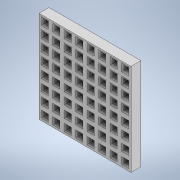
# Autodesk Inventor part: StandMatrix
Saved by Autodesk Inventor 2020.1 (Build 241239000, 239)
## iProperties
Created: 2019-09-02
Part Number: StandMatrix
Material: Generic
Document SubType Name: Modeling
Designer: matteo.spadetto-1
Density: 1 g/cm^3
Appearance: Default
Author: matteo.spadetto-1
Autodesk Inventor part; units mm, degrees
(part 1 of 2)
ref_plane "YZ Plane" through (0, 0, 0) normal (1, 0, 0) x (0, 1, 0)
ref_plane "XZ Plane" through (0, 0, 0) normal (0, 1, 0) x (-1, 0, 0)
ref_plane "XY Plane" through (0, 0, 0) normal (0, 0, 1) x (1, 0, 0)
sketch "Sketch1" plane through (0, 0, 0) normal (0, 0, 1) x (1, 0, 0)
  line L0 (1.062, 57.938) -> (1.062, 63.938)
  line L1 (1.062, 63.938) -> (7.062, 63.938)
  line L2 (7.062, 63.938) -> (7.062, 57.938)
  line L3 (7.062, 57.938) -> (1.062, 57.938)
  line L4 (17.31, 57.938) -> (23.31, 57.938)
  line L5 (23.31, 57.938) -> (23.31, 63.938)
  line L6 (23.31, 63.938) -> (17.31, 63.938)
  line L7 (17.31, 63.938) -> (17.31, 57.938)
  line L8 (9.186, 57.938) -> (15.186, 57.938)
  line L9 (15.186, 57.938) -> (15.186, 63.938)
  line L10 (15.186, 63.938) -> (9.186, 63.938)
  line L11 (9.186, 63.938) -> (9.186, 57.938)
  line L12 (25.434, 57.938) -> (31.434, 57.938)
  line L13 (31.434, 57.938) -> (31.434, 63.938)
  line L14 (31.434, 63.938) -> (25.434, 63.938)
  line L15 (25.434, 63.938) -> (25.434, 57.938)
  line L16 (33.558, 57.938) -> (39.558, 57.938)
  line L17 (39.558, 57.938) -> (39.558, 63.938)
  line L18 (39.558, 63.938) -> (33.558, 63.938)
  line L19 (33.558, 63.938) -> (33.558, 57.938)
  line L20 (47.682, 57.938) -> (41.682, 57.938)
  line L21 (41.682, 57.938) -> (41.682, 63.938)
  line L22 (41.682, 63.938) -> (47.682, 63.938)
  line L23 (47.682, 63.938) -> (47.682, 57.938)
  line L24 (55.806, 57.938) -> (49.806, 57.938)
  line L25 (49.806, 57.938) -> (49.806, 63.938)
  line L26 (49.806, 63.938) -> (55.806, 63.938)
  line L27 (55.806, 63.938) -> (55.806, 57.938)
  line L28 (63.93, 57.938) -> (57.93, 57.938)
  line L29 (57.93, 57.938) -> (57.93, 63.938)
  line L30 (57.93, 63.938) -> (63.93, 63.938)
  line L31 (63.93, 63.938) -> (63.93, 57.938)
  line L32 (1.062, 49.814) -> (1.062, 55.814)
  line L33 (1.062, 55.814) -> (7.062, 55.814)
  line L34 (7.062, 55.814) -> (7.062, 49.814)
  line L35 (7.062, 49.814) -> (1.062, 49.814)
  line L36 (9.186, 49.814) -> (15.186, 49.814)
  line L37 (15.186, 49.814) -> (15.186, 55.814)
  line L38 (15.186, 55.814) -> (9.186, 55.814)
  line L39 (9.186, 55.814) -> (9.186, 49.814)
  line L40 (17.31, 49.814) -> (17.31, 55.814)
  line L41 (17.31, 55.814) -> (23.31, 55.814)
  line L42 (23.31, 55.814) -> (23.31, 49.814)
  line L43 (23.31, 49.814) -> (17.31, 49.814)
  line L44 (25.434, 55.814) -> (31.434, 55.814)
  line L45 (31.434, 55.814) -> (31.434, 49.814)
  line L46 (31.434, 49.814) -> (25.434, 49.814)
  line L47 (33.558, 55.814) -> (39.558, 55.814)
  line L48 (39.558, 55.814) -> (39.558, 49.814)
  line L49 (39.558, 49.814) -> (33.558, 49.814)
  line L50 (47.682, 49.814) -> (41.682, 49.814)
  line L51 (41.682, 49.814) -> (41.682, 55.814)
  line L52 (41.682, 55.814) -> (47.682, 55.814)
  line L53 (47.682, 55.814) -> (47.682, 49.814)
  line L54 (49.806, 49.814) -> (55.806, 49.814)
  line L55 (55.806, 49.814) -> (55.806, 55.814)
  line L56 (55.806, 55.814) -> (49.806, 55.814)
  line L57 (49.806, 55.814) -> (49.806, 49.814)
  line L58 (63.93, 49.814) -> (57.93, 49.814)
  line L59 (57.93, 49.814) -> (57.93, 55.814)
  line L60 (57.93, 55.814) -> (63.93, 55.814)
  line L61 (63.93, 55.814) -> (63.93, 49.814)
  line L62 (1.062, 41.69) -> (7.062, 41.69)
  line L63 (7.062, 41.69) -> (7.062, 47.69)
  line L64 (7.062, 47.69) -> (1.062, 47.69)
  line L65 (1.062, 47.69) -> (1.062, 41.69)
  line L66 (9.186, 41.69) -> (9.186, 47.69)
  line L67 (9.186, 47.69) -> (15.186, 47.69)
  line L68 (15.186, 47.69) -> (15.186, 41.69)
  line L69 (15.186, 41.69) -> (9.186, 41.69)
  line L70 (23.31, 41.69) -> (23.31, 47.69)
  line L71 (23.31, 47.69) -> (17.31, 47.69)
  line L72 (17.31, 47.69) -> (17.31, 41.69)
  line L73 (17.31, 41.69) -> (23.31, 41.69)
  line L74 (31.434, 41.69) -> (25.434, 41.69)
  line L75 (25.434, 41.69) -> (25.434, 47.69)
  line L76 (25.434, 47.69) -> (31.434, 47.69)
  line L77 (31.434, 47.69) -> (31.434, 41.69)
  line L78 (39.558, 41.69) -> (33.558, 41.69)
  line L79 (33.558, 41.69) -> (33.558, 47.69)
  line L80 (33.558, 47.69) -> (39.558, 47.69)
  line L81 (39.558, 47.69) -> (39.558, 41.69)
  line L82 (47.682, 41.69) -> (47.682, 47.69)
  line L83 (47.682, 47.69) -> (41.682, 47.69)
  line L84 (41.682, 47.69) -> (41.682, 41.69)
  line L85 (41.682, 41.69) -> (47.682, 41.69)
  line L86 (55.806, 41.69) -> (55.806, 47.69)
  line L87 (55.806, 47.69) -> (49.806, 47.69)
  line L88 (49.806, 47.69) -> (49.806, 41.69)
  line L89 (49.806, 41.69) -> (55.806, 41.69)
  line L90 (63.93, 41.69) -> (63.93, 47.69)
  line L91 (63.93, 47.69) -> (57.93, 47.69)
  line L92 (57.93, 47.69) -> (57.93, 41.69)
  line L93 (57.93, 41.69) -> (63.93, 41.69)
  line L94 (7.062, 33.566) -> (1.062, 33.566)
  line L95 (1.062, 33.566) -> (1.062, 39.566)
  line L96 (1.062, 39.566) -> (7.062, 39.566)
  line L97 (7.062, 39.566) -> (7.062, 33.566)
  line L98 (15.186, 33.566) -> (15.186, 39.566)
  line L99 (15.186, 39.566) -> (9.186, 39.566)
  line L100 (9.186, 39.566) -> (9.186, 33.566)
  line L101 (9.186, 33.566) -> (15.186, 33.566)
  line L102 (17.31, 33.566) -> (23.31, 33.566)
  line L103 (23.31, 33.566) -> (23.31, 39.566)
  line L104 (23.31, 39.566) -> (17.31, 39.566)
  line L105 (17.31, 39.566) -> (17.31, 33.566)
  line L106 (25.434, 33.566) -> (31.434, 33.566)
  line L107 (31.434, 33.566) -> (31.434, 39.566)
  line L108 (31.434, 39.566) -> (25.434, 39.566)
  line L109 (25.434, 39.566) -> (25.434, 33.566)
  line L110 (39.558, 33.566) -> (33.558, 33.566)
  line L111 (33.558, 33.566) -> (33.558, 39.566)
  line L112 (33.558, 39.566) -> (39.558, 39.566)
  line L113 (39.558, 39.566) -> (39.558, 33.566)
  line L114 (41.682, 33.566) -> (41.682, 39.566)
  line L115 (41.682, 39.566) -> (47.682, 39.566)
  line L116 (47.682, 39.566) -> (47.682, 33.566)
  line L117 (47.682, 33.566) -> (41.682, 33.566)
  line L118 (55.806, 33.566) -> (49.806, 33.566)
  line L119 (49.806, 33.566) -> (49.806, 39.566)
  line L120 (49.806, 39.566) -> (55.806, 39.566)
  line L121 (55.806, 39.566) -> (55.806, 33.566)
  line L122 (63.93, 33.566) -> (57.93, 33.566)
  line L123 (57.93, 33.566) -> (57.93, 39.566)
  line L124 (57.93, 39.566) -> (63.93, 39.566)
  line L125 (63.93, 39.566) -> (63.93, 33.566)
  line L126 (25.434, 49.814) -> (25.434, 55.814)
  line L127 (33.558, 55.814) -> (33.558, 49.814)
  line L128 (1.062, 7.062) -> (1.062, 1.062)
  line L129 (1.062, 1.062) -> (7.062, 1.062)
  line L130 (7.062, 1.062) -> (7.062, 7.062)
  line L131 (7.062, 7.062) -> (1.062, 7.062)
  line L132 (17.31, 7.062) -> (23.31, 7.062)
  line L133 (23.31, 7.062) -> (23.31, 1.062)
  line L134 (23.31, 1.062) -> (17.31, 1.062)
  line L135 (17.31, 1.062) -> (17.31, 7.062)
  line L136 (9.186, 7.062) -> (15.186, 7.062)
  line L137 (15.186, 7.062) -> (15.186, 1.062)
  line L138 (15.186, 1.062) -> (9.186, 1.062)
  line L139 (9.186, 1.062) -> (9.186, 7.062)
  line L140 (25.434, 7.062) -> (31.434, 7.062)
  line L141 (31.434, 7.062) -> (31.434, 1.062)
  line L142 (31.434, 1.062) -> (25.434, 1.062)
  line L143 (25.434, 1.062) -> (25.434, 7.062)
  line L144 (33.558, 7.062) -> (39.558, 7.062)
  line L145 (39.558, 7.062) -> (39.558, 1.062)
  line L146 (39.558, 1.062) -> (33.558, 1.062)
  line L147 (33.558, 1.062) -> (33.558, 7.062)
  line L148 (47.682, 7.062) -> (41.682, 7.062)
  line L149 (41.682, 7.062) -> (41.682, 1.062)
  line L150 (41.682, 1.062) -> (47.682, 1.062)
  line L151 (47.682, 1.062) -> (47.682, 7.062)
  line L152 (55.806, 7.062) -> (49.806, 7.062)
  line L153 (49.806, 7.062) -> (49.806, 1.062)
  line L154 (49.806, 1.062) -> (55.806, 1.062)
  line L155 (55.806, 1.062) -> (55.806, 7.062)
  line L156 (63.93, 7.062) -> (57.93, 7.062)
  line L157 (57.93, 7.062) -> (57.93, 1.062)
  line L158 (57.93, 1.062) -> (63.93, 1.062)
  line L159 (63.93, 1.062) -> (63.93, 7.062)
  line L160 (1.062, 15.186) -> (1.062, 9.186)
  line L161 (1.062, 9.186) -> (7.062, 9.186)
  line L162 (7.062, 9.186) -> (7.062, 15.186)
  line L163 (7.062, 15.186) -> (1.062, 15.186)
  line L164 (9.186, 15.186) -> (15.186, 15.186)
  line L165 (15.186, 15.186) -> (15.186, 9.186)
  line L166 (15.186, 9.186) -> (9.186, 9.186)
  line L167 (9.186, 9.186) -> (9.186, 15.186)
  line L168 (17.31, 15.186) -> (17.31, 9.186)
  line L169 (17.31, 9.186) -> (23.31, 9.186)
  line L170 (23.31, 9.186) -> (23.31, 15.186)
  line L171 (23.31, 15.186) -> (17.31, 15.186)
  line L172 (25.434, 9.186) -> (31.434, 9.186)
  line L173 (31.434, 9.186) -> (31.434, 15.186)
  line L174 (31.434, 15.186) -> (25.434, 15.186)
  line L175 (33.558, 9.186) -> (39.558, 9.186)
  line L176 (39.558, 9.186) -> (39.558, 15.186)
  line L177 (39.558, 15.186) -> (33.558, 15.186)
  line L178 (47.682, 15.186) -> (41.682, 15.186)
  line L179 (41.682, 15.186) -> (41.682, 9.186)
  line L180 (41.682, 9.186) -> (47.682, 9.186)
  line L181 (47.682, 9.186) -> (47.682, 15.186)
  line L182 (49.806, 15.186) -> (55.806, 15.186)
  line L183 (55.806, 15.186) -> (55.806, 9.186)
  line L184 (55.806, 9.186) -> (49.806, 9.186)
  line L185 (49.806, 9.186) -> (49.806, 15.186)
  line L186 (63.93, 15.186) -> (57.93, 15.186)
  line L187 (57.93, 15.186) -> (57.93, 9.186)
  line L188 (57.93, 9.186) -> (63.93, 9.186)
  line L189 (63.93, 9.186) -> (63.93, 15.186)
  line L190 (1.062, 23.31) -> (7.062, 23.31)
  line L191 (7.062, 23.31) -> (7.062, 17.31)
  line L192 (7.062, 17.31) -> (1.062, 17.31)
  line L193 (1.062, 17.31) -> (1.062, 23.31)
  line L194 (9.186, 23.31) -> (9.186, 17.31)
  line L195 (9.186, 17.31) -> (15.186, 17.31)
  line L196 (15.186, 17.31) -> (15.186, 23.31)
  line L197 (15.186, 23.31) -> (9.186, 23.31)
  line L198 (23.31, 23.31) -> (23.31, 17.31)
  line L199 (23.31, 17.31) -> (17.31, 17.31)
  line L200 (17.31, 17.31) -> (17.31, 23.31)
  line L201 (17.31, 23.31) -> (23.31, 23.31)
  line L202 (31.434, 23.31) -> (25.434, 23.31)
  line L203 (25.434, 23.31) -> (25.434, 17.31)
  line L204 (25.434, 17.31) -> (31.434, 17.31)
  line L205 (31.434, 17.31) -> (31.434, 23.31)
  line L206 (39.558, 23.31) -> (33.558, 23.31)
  line L207 (33.558, 23.31) -> (33.558, 17.31)
  line L208 (33.558, 17.31) -> (39.558, 17.31)
  line L209 (39.558, 17.31) -> (39.558, 23.31)
  line L210 (47.682, 23.31) -> (47.682, 17.31)
  line L211 (47.682, 17.31) -> (41.682, 17.31)
  line L212 (41.682, 17.31) -> (41.682, 23.31)
  line L213 (41.682, 23.31) -> (47.682, 23.31)
  line L214 (55.806, 23.31) -> (55.806, 17.31)
  line L215 (55.806, 17.31) -> (49.806, 17.31)
  line L216 (49.806, 17.31) -> (49.806, 23.31)
  line L217 (49.806, 23.31) -> (55.806, 23.31)
  line L218 (63.93, 23.31) -> (63.93, 17.31)
  line L219 (63.93, 17.31) -> (57.93, 17.31)
  line L220 (57.93, 17.31) -> (57.93, 23.31)
  line L221 (57.93, 23.31) -> (63.93, 23.31)
  line L222 (7.062, 31.434) -> (1.062, 31.434)
  line L223 (1.062, 31.434) -> (1.062, 25.434)
  line L224 (1.062, 25.434) -> (7.062, 25.434)
  line L225 (7.062, 25.434) -> (7.062, 31.434)
  line L226 (15.186, 31.434) -> (15.186, 25.434)
  line L227 (15.186, 25.434) -> (9.186, 25.434)
  line L228 (9.186, 25.434) -> (9.186, 31.434)
  line L229 (9.186, 31.434) -> (15.186, 31.434)
  line L230 (17.31, 31.434) -> (23.31, 31.434)
  line L231 (23.31, 31.434) -> (23.31, 25.434)
  line L232 (23.31, 25.434) -> (17.31, 25.434)
  line L233 (17.31, 25.434) -> (17.31, 31.434)
  line L234 (25.434, 31.434) -> (31.434, 31.434)
  line L235 (31.434, 31.434) -> (31.434, 25.434)
  line L236 (31.434, 25.434) -> (25.434, 25.434)
  line L237 (25.434, 25.434) -> (25.434, 31.434)
  line L238 (39.558, 31.434) -> (33.558, 31.434)
  line L239 (33.558, 31.434) -> (33.558, 25.434)
  line L240 (33.558, 25.434) -> (39.558, 25.434)
  line L241 (39.558, 25.434) -> (39.558, 31.434)
  line L242 (41.682, 31.434) -> (41.682, 25.434)
  line L243 (41.682, 25.434) -> (47.682, 25.434)
  line L244 (47.682, 25.434) -> (47.682, 31.434)
  line L245 (47.682, 31.434) -> (41.682, 31.434)
  line L246 (55.806, 31.434) -> (49.806, 31.434)
  line L247 (49.806, 31.434) -> (49.806, 25.434)
  line L248 (49.806, 25.434) -> (55.806, 25.434)
  line L249 (55.806, 25.434) -> (55.806, 31.434)
  line L250 (63.93, 31.434) -> (57.93, 31.434)
  line L251 (57.93, 31.434) -> (57.93, 25.434)
  line L252 (57.93, 25.434) -> (63.93, 25.434)
  line L253 (63.93, 25.434) -> (63.93, 31.434)
  line L254 (25.434, 15.186) -> (25.434, 9.186)
  line L255 (33.558, 9.186) -> (33.558, 15.186)
  line L256 (0, 65) -> (0, 0)
  line L257 (0, 0) -> (65, 0)
  line L258 (0, 65) -> (65, 65)
  line L259 (65, 65) -> (65, 0)
  line L260 (2.062, 62.938) -> (2.062, 58.938)
  line L261 (2.062, 58.938) -> (6.062, 58.938)
  line L262 (6.062, 58.938) -> (6.062, 62.938)
  line L263 (6.062, 62.938) -> (2.062, 62.938)
  line L264 (2.062, 54.814) -> (2.062, 50.814)
  line L265 (6.062, 54.814) -> (2.062, 54.814)
  line L266 (6.062, 50.814) -> (6.062, 54.814)
  line L267 (2.062, 50.814) -> (6.062, 50.814)
  line L268 (2.062, 46.69) -> (2.062, 42.69)
  line L269 (6.062, 46.69) -> (2.062, 46.69)
  line L270 (6.062, 42.69) -> (6.062, 46.69)
  line L271 (2.062, 42.69) -> (6.062, 42.69)
  line L272 (2.062, 38.566) -> (2.062, 34.566)
  line L273 (6.062, 38.566) -> (2.062, 38.566)
  line L274 (6.062, 34.566) -> (6.062, 38.566)
  line L275 (2.062, 34.566) -> (6.062, 34.566)
  line L276 (2.062, 30.442) -> (2.062, 26.442)
  line L277 (6.062, 30.442) -> (2.062, 30.442)
  line L278 (6.062, 26.442) -> (6.062, 30.442)
  line L279 (2.062, 26.442) -> (6.062, 26.442)
  line L280 (2.062, 22.318) -> (2.062, 18.318)
  line L281 (6.062, 22.318) -> (2.062, 22.318)
  line L282 (6.062, 18.318) -> (6.062, 22.318)
  line L283 (2.062, 18.318) -> (6.062, 18.318)
  line L284 (2.062, 14.194) -> (2.062, 10.194)
  line L285 (6.062, 14.194) -> (2.062, 14.194)
  line L286 (6.062, 10.194) -> (6.062, 14.194)
  line L287 (2.062, 10.194) -> (6.062, 10.194)
  line L288 (2.062, 6.07) -> (2.062, 2.07)
  line L289 (6.062, 6.07) -> (2.062, 6.07)
  line L290 (6.062, 2.07) -> (6.062, 6.07)
  line L291 (2.062, 2.07) -> (6.062, 2.07)
  line L292 (10.186, 62.938) -> (10.186, 58.938)
  line L293 (14.186, 62.938) -> (10.186, 62.938)
  line L294 (14.186, 58.938) -> (14.186, 62.938)
  line L295 (10.186, 58.938) -> (14.186, 58.938)
  line L296 (10.186, 54.814) -> (10.186, 50.814)
  line L297 (14.186, 54.814) -> (10.186, 54.814)
  line L298 (14.186, 50.814) -> (14.186, 54.814)
  line L299 (10.186, 50.814) -> (14.186, 50.814)
  line L300 (10.186, 46.69) -> (10.186, 42.69)
  line L301 (14.186, 46.69) -> (10.186, 46.69)
  line L302 (14.186, 42.69) -> (14.186, 46.69)
  line L303 (10.186, 42.69) -> (14.186, 42.69)
  line L304 (10.186, 38.566) -> (10.186, 34.566)
  line L305 (14.186, 38.566) -> (10.186, 38.566)
  line L306 (14.186, 34.566) -> (14.186, 38.566)
  line L307 (10.186, 34.566) -> (14.186, 34.566)
  line L308 (10.186, 30.442) -> (10.186, 26.442)
  line L309 (14.186, 30.442) -> (10.186, 30.442)
  line L310 (14.186, 26.442) -> (14.186, 30.442)
  line L311 (10.186, 26.442) -> (14.186, 26.442)
  line L312 (10.186, 22.318) -> (10.186, 18.318)
  line L313 (14.186, 22.318) -> (10.186, 22.318)
  line L314 (14.186, 18.318) -> (14.186, 22.318)
  line L315 (10.186, 18.318) -> (14.186, 18.318)
  line L316 (10.186, 14.194) -> (10.186, 10.194)
  line L317 (14.186, 14.194) -> (10.186, 14.194)
  line L318 (14.186, 10.194) -> (14.186, 14.194)
  line L319 (10.186, 10.194) -> (14.186, 10.194)
  line L320 (10.186, 6.07) -> (10.186, 2.07)
  line L321 (14.186, 6.07) -> (10.186, 6.07)
  line L322 (14.186, 2.07) -> (14.186, 6.07)
  line L323 (10.186, 2.07) -> (14.186, 2.07)
  line L324 (18.31, 62.938) -> (18.31, 58.938)
  line L325 (22.31, 62.938) -> (18.31, 62.938)
  line L326 (22.31, 58.938) -> (22.31, 62.938)
  line L327 (18.31, 58.938) -> (22.31, 58.938)
  line L328 (18.31, 54.814) -> (18.31, 50.814)
  line L329 (22.31, 54.814) -> (18.31, 54.814)
  line L330 (22.31, 50.814) -> (22.31, 54.814)
  line L331 (18.31, 50.814) -> (22.31, 50.814)
  line L332 (18.31, 46.69) -> (18.31, 42.69)
  line L333 (22.31, 46.69) -> (18.31, 46.69)
  line L334 (22.31, 42.69) -> (22.31, 46.69)
  line L335 (18.31, 42.69) -> (22.31, 42.69)
  line L336 (18.31, 38.566) -> (18.31, 34.566)
  line L337 (22.31, 38.566) -> (18.31, 38.566)
  line L338 (22.31, 34.566) -> (22.31, 38.566)
  line L339 (18.31, 34.566) -> (22.31, 34.566)
  line L340 (18.31, 30.442) -> (18.31, 26.442)
  line L341 (22.31, 30.442) -> (18.31, 30.442)
  line L342 (22.31, 26.442) -> (22.31, 30.442)
  line L343 (18.31, 26.442) -> (22.31, 26.442)
  line L344 (18.31, 22.318) -> (18.31, 18.318)
  line L345 (22.31, 22.318) -> (18.31, 22.318)
  line L346 (22.31, 18.318) -> (22.31, 22.318)
  line L347 (18.31, 18.318) -> (22.31, 18.318)
  line L348 (18.31, 14.194) -> (18.31, 10.194)
  line L349 (22.31, 14.194) -> (18.31, 14.194)
  line L350 (22.31, 10.194) -> (22.31, 14.194)
  line L351 (18.31, 10.194) -> (22.31, 10.194)
  line L352 (18.31, 6.07) -> (18.31, 2.07)
  line L353 (22.31, 6.07) -> (18.31, 6.07)
  line L354 (22.31, 2.07) -> (22.31, 6.07)
  line L355 (18.31, 2.07) -> (22.31, 2.07)
  line L356 (26.434, 62.938) -> (26.434, 58.938)
  line L357 (30.434, 62.938) -> (26.434, 62.938)
  line L358 (30.434, 58.938) -> (30.434, 62.938)
  line L359 (26.434, 58.938) -> (30.434, 58.938)
  line L360 (26.434, 54.814) -> (26.434, 50.814)
  line L361 (30.434, 54.814) -> (26.434, 54.814)
  line L362 (30.434, 50.814) -> (30.434, 54.814)
  line L363 (26.434, 50.814) -> (30.434, 50.814)
  line L364 (26.434, 46.69) -> (26.434, 42.69)
  line L365 (30.434, 46.69) -> (26.434, 46.69)
  line L366 (30.434, 42.69) -> (30.434, 46.69)
  line L367 (26.434, 42.69) -> (30.434, 42.69)
  line L368 (26.434, 38.566) -> (26.434, 34.566)
  line L369 (30.434, 38.566) -> (26.434, 38.566)
  line L370 (30.434, 34.566) -> (30.434, 38.566)
  line L371 (26.434, 34.566) -> (30.434, 34.566)
  line L372 (26.434, 30.442) -> (26.434, 26.442)
  line L373 (30.434, 30.442) -> (26.434, 30.442)
  line L374 (30.434, 26.442) -> (30.434, 30.442)
  line L375 (26.434, 26.442) -> (30.434, 26.442)
  line L376 (26.434, 22.318) -> (26.434, 18.318)
  line L377 (30.434, 22.318) -> (26.434, 22.318)
  line L378 (30.434, 18.318) -> (30.434, 22.318)
  line L379 (26.434, 18.318) -> (30.434, 18.318)
  line L380 (26.434, 14.194) -> (26.434, 10.194)
  line L381 (30.434, 14.194) -> (26.434, 14.194)
  line L382 (30.434, 10.194) -> (30.434, 14.194)
  line L383 (26.434, 10.194) -> (30.434, 10.194)
  line L384 (26.434, 6.07) -> (26.434, 2.07)
  line L385 (30.434, 6.07) -> (26.434, 6.07)
  line L386 (30.434, 2.07) -> (30.434, 6.07)
  line L387 (26.434, 2.07) -> (30.434, 2.07)
  line L388 (34.558, 62.938) -> (34.558, 58.938)
  line L389 (38.558, 62.938) -> (34.558, 62.938)
  line L390 (38.558, 58.938) -> (38.558, 62.938)
  line L391 (34.558, 58.938) -> (38.558, 58.938)
  line L392 (34.558, 54.814) -> (34.558, 50.814)
  line L393 (38.558, 54.814) -> (34.558, 54.814)
  line L394 (38.558, 50.814) -> (38.558, 54.814)
  line L395 (34.558, 50.814) -> (38.558, 50.814)
  line L396 (34.558, 46.69) -> (34.558, 42.69)
  line L397 (38.558, 46.69) -> (34.558, 46.69)
  line L398 (38.558, 42.69) -> (38.558, 46.69)
  line L399 (34.558, 42.69) -> (38.558, 42.69)
  line L400 (34.558, 38.566) -> (34.558, 34.566)
  line L401 (38.558, 38.566) -> (34.558, 38.566)
  line L402 (38.558, 34.566) -> (38.558, 38.566)
  line L403 (34.558, 34.566) -> (38.558, 34.566)
  line L404 (34.558, 30.442) -> (34.558, 26.442)
  line L405 (38.558, 30.442) -> (34.558, 30.442)
  line L406 (38.558, 26.442) -> (38.558, 30.442)
  line L407 (34.558, 26.442) -> (38.558, 26.442)
  line L408 (34.558, 22.318) -> (34.558, 18.318)
  line L409 (38.558, 22.318) -> (34.558, 22.318)
  line L410 (38.558, 18.318) -> (38.558, 22.318)
  line L411 (34.558, 18.318) -> (38.558, 18.318)
  line L412 (34.558, 14.194) -> (34.558, 10.194)
  line L413 (38.558, 14.194) -> (34.558, 14.194)
  line L414 (38.558, 10.194) -> (38.558, 14.194)
  line L415 (34.558, 10.194) -> (38.558, 10.194)
  line L416 (34.558, 6.07) -> (34.558, 2.07)
  line L417 (38.558, 6.07) -> (34.558, 6.07)
  line L418 (38.558, 2.07) -> (38.558, 6.07)
  line L419 (34.558, 2.07) -> (38.558, 2.07)
  line L420 (42.682, 62.938) -> (42.682, 58.938)
  line L421 (46.682, 62.938) -> (42.682, 62.938)
  line L422 (46.682, 58.938) -> (46.682, 62.938)
  line L423 (42.682, 58.938) -> (46.682, 58.938)
  line L424 (42.682, 54.814) -> (42.682, 50.814)
  line L425 (46.682, 54.814) -> (42.682, 54.814)
  line L426 (46.682, 50.814) -> (46.682, 54.814)
  line L427 (42.682, 50.814) -> (46.682, 50.814)
  line L428 (42.682, 46.69) -> (42.682, 42.69)
  line L429 (46.682, 46.69) -> (42.682, 46.69)
  line L430 (46.682, 42.69) -> (46.682, 46.69)
  line L431 (42.682, 42.69) -> (46.682, 42.69)
  line L432 (42.682, 38.566) -> (42.682, 34.566)
  line L433 (46.682, 38.566) -> (42.682, 38.566)
  line L434 (46.682, 34.566) -> (46.682, 38.566)
  line L435 (42.682, 34.566) -> (46.682, 34.566)
  line L436 (42.682, 30.442) -> (42.682, 26.442)
  line L437 (46.682, 30.442) -> (42.682, 30.442)
  line L438 (46.682, 26.442) -> (46.682, 30.442)
  line L439 (42.682, 26.442) -> (46.682, 26.442)
  line L440 (42.682, 22.318) -> (42.682, 18.318)
  line L441 (46.682, 22.318) -> (42.682, 22.318)
  line L442 (46.682, 18.318) -> (46.682, 22.318)
  line L443 (42.682, 18.318) -> (46.682, 18.318)
  line L444 (42.682, 14.194) -> (42.682, 10.194)
  line L445 (46.682, 14.194) -> (42.682, 14.194)
  line L446 (46.682, 10.194) -> (46.682, 14.194)
  line L447 (42.682, 10.194) -> (46.682, 10.194)
  line L448 (42.682, 6.07) -> (42.682, 2.07)
  line L449 (46.682, 6.07) -> (42.682, 6.07)
  line L450 (46.682, 2.07) -> (46.682, 6.07)
  line L451 (42.682, 2.07) -> (46.682, 2.07)
  line L452 (50.806, 62.938) -> (50.806, 58.938)
  line L453 (54.806, 62.938) -> (50.806, 62.938)
  line L454 (54.806, 58.938) -> (54.806, 62.938)
  line L455 (50.806, 58.938) -> (54.806, 58.938)
  line L456 (50.806, 54.814) -> (50.806, 50.814)
  line L457 (54.806, 54.814) -> (50.806, 54.814)
  line L458 (54.806, 50.814) -> (54.806, 54.814)
  line L459 (50.806, 50.814) -> (54.806, 50.814)
  line L460 (50.806, 46.69) -> (50.806, 42.69)
  line L461 (54.806, 46.69) -> (50.806, 46.69)
  line L462 (54.806, 42.69) -> (54.806, 46.69)
  line L463 (50.806, 42.69) -> (54.806, 42.69)
  line L464 (50.806, 38.566) -> (50.806, 34.566)
  line L465 (54.806, 38.566) -> (50.806, 38.566)
  line L466 (54.806, 34.566) -> (54.806, 38.566)
  line L467 (50.806, 34.566) -> (54.806, 34.566)
  line L468 (50.806, 30.442) -> (50.806, 26.442)
  line L469 (54.806, 30.442) -> (50.806, 30.442)
  line L470 (54.806, 26.442) -> (54.806, 30.442)
  line L471 (50.806, 26.442) -> (54.806, 26.442)
  line L472 (50.806, 22.318) -> (50.806, 18.318)
  line L473 (54.806, 22.318) -> (50.806, 22.318)
  line L474 (54.806, 18.318) -> (54.806, 22.318)
  line L475 (50.806, 18.318) -> (54.806, 18.318)
  line L476 (50.806, 14.194) -> (50.806, 10.194)
  line L477 (54.806, 14.194) -> (50.806, 14.194)
  line L478 (54.806, 10.194) -> (54.806, 14.194)
  line L479 (50.806, 10.194) -> (54.806, 10.194)
  line L480 (50.806, 6.07) -> (50.806, 2.07)
  line L481 (54.806, 6.07) -> (50.806, 6.07)
  line L482 (54.806, 2.07) -> (54.806, 6.07)
  line L483 (50.806, 2.07) -> (54.806, 2.07)
  line L484 (58.93, 62.938) -> (58.93, 58.938)
  line L485 (62.93, 62.938) -> (58.93, 62.938)
  line L486 (62.93, 58.938) -> (62.93, 62.938)
  line L487 (58.93, 58.938) -> (62.93, 58.938)
  line L488 (58.93, 54.814) -> (58.93, 50.814)
  line L489 (62.93, 54.814) -> (58.93, 54.814)
  line L490 (62.93, 50.814) -> (62.93, 54.814)
  line L491 (58.93, 50.814) -> (62.93, 50.814)
  line L492 (58.93, 46.69) -> (58.93, 42.69)
  line L493 (62.93, 46.69) -> (58.93, 46.69)
  line L494 (62.93, 42.69) -> (62.93, 46.69)
  line L495 (58.93, 42.69) -> (62.93, 42.69)
  line L496 (58.93, 38.566) -> (58.93, 34.566)
  line L497 (62.93, 38.566) -> (58.93, 38.566)
  line L498 (62.93, 34.566) -> (62.93, 38.566)
  line L499 (58.93, 34.566) -> (62.93, 34.566)
  line L500 (58.93, 30.442) -> (58.93, 26.442)
  line L501 (62.93, 30.442) -> (58.93, 30.442)
  line L502 (62.93, 26.442) -> (62.93, 30.442)
  line L503 (58.93, 26.442) -> (62.93, 26.442)
  line L504 (58.93, 22.318) -> (58.93, 18.318)
  line L505 (62.93, 22.318) -> (58.93, 22.318)
  line L506 (62.93, 18.318) -> (62.93, 22.318)
  line L507 (58.93, 18.318) -> (62.93, 18.318)
  line L508 (58.93, 14.194) -> (58.93, 10.194)
  line L509 (62.93, 14.194) -> (58.93, 14.194)
  line L510 (62.93, 10.194) -> (62.93, 14.194)
  line L511 (58.93, 10.194) -> (62.93, 10.194)
  line L512 (58.93, 6.07) -> (58.93, 2.07)
  line L513 (62.93, 6.07) -> (58.93, 6.07)
  line L514 (62.93, 2.07) -> (62.93, 6.07)
  line L515 (58.93, 2.07) -> (62.93, 2.07)
  dimension "d36" = 1
  dimension "d41" = 8.124
  dimension "d44" = 8.124
  dimension "d64" = 4
  dimension "d65" = 4
  constraints: 1032 end point, 2 collinear, 1 horizontal, 1 vertical, 505 other
  measures "d36" distance between parallel lines of L0 L260
  measures "d41" distance of L260.start L264.start
  measures "d44" distance of L260.start L292.start
  measures "d64" distance of L293.start L292.start
  measures "d65" distance of L292.end L294.start
extrude "Extrusion1" add sketch "Sketch1" along normal blind 7 contours L258 L259 L257 L256
extrude "Extrusion2" add sketch "Sketch1" along normal blind 3.5 contours L0 L1 L2 L3 | L7 L6 L5 L4 | L11 L10 L9 L8 | L15 L14 L13 L12 | L19 L18 L17 L16 | L20 L21 L22 L23 | L24 L25 L26 L27 | L28 L29 L30 L31 | L32 L33 L34 L35 | L39 L38 L37 L36 | L40 L41 L42 L43 | L44 L45 L46 L126 | L47 L48 L49 L127 | L50 L51 L52 L53 | L57 L56 L55 L54 | L58 L59 L60 L61 | L65 L64 L63 L62 | L66 L67 L68 L69 | L73 L72 L71 L70 | L74 L75 L76 L77 | L78 L79 L80 L81 | L85 L84 L83 L82 | L89 L88 L87 L86 | L93 L92 L91 L90 | L94 L95 L96 L97 | L101 L100 L99 L98 | L105 L104 L103 L102 | L109 L108 L107 L106 | L110 L111 L112 L113 | L114 L115 L116 L117 | L118 L119 L120 L121 | L122 L123 L124 L125 | L131 L130 L129 L128 | L132 L133 L134 L135 | L136 L137 L138 L139 | L140 L141 L142 L143 | L144 L145 L146 L147 | L151 L150 L149 L148 | L155 L154 L153 L152 | L159 L158 L157 L156 | L163 L162 L161 L160 | L164 L165 L166 L167 | L171 L170 L169 L168 | L254 L174 L173 L172 | L255 L177 L176 L175 | L181 L180 L179 L178 | L182 L183 L184 L185 | L189 L188 L187 L186 | L190 L191 L192 L193 | L197 L196 L195 L194 | L198 L199 L200 L201 | L205 L204 L203 L202 | L209 L208 L207 L206 | L210 L211 L212 L213 | L214 L215 L216 L217 | L218 L219 L220 L221 | L225 L224 L223 L222 | L226 L227 L228 L229 | L230 L231 L232 L233 | L234 L235 L236 L237 | L241 L240 L239 L238 | L245 L244 L243 L242 | L249 L248 L247 L246 | L253 L252 L251 L250 | L258 L259 L257 L256 | L473 L474 L475 L472
extrude "Extrusion3" cut sketch "Sketch1" along normal blind 3.5 contours L473 L474 L475 L472
extrude "Extrusion4" cut sketch "Sketch1" along normal blind 2.5 contours L0 L1 L2 L3 | L7 L6 L5 L4 | L11 L10 L9 L8 | L15 L14 L13 L12 | L19 L18 L17 L16 | L20 L21 L22 L23 | L24 L25 L26 L27 | L28 L29 L30 L31 | L32 L33 L34 L35 | L39 L38 L37 L36 | L40 L41 L42 L43 | L44 L45 L46 L126 | L47 L48 L49 L127 | L50 L51 L52 L53 | L57 L56 L55 L54 | L58 L59 L60 L61 | L65 L64 L63 L62 | L66 L67 L68 L69 | L73 L72 L71 L70 | L74 L75 L76 L77 | L78 L79 L80 L81 | L85 L84 L83 L82 | L89 L88 L87 L86 | L93 L92 L91 L90 | L94 L95 L96 L97 | L101 L100 L99 L98 | L105 L104 L103 L102 | L109 L108 L107 L106 | L110 L111 L112 L113 | L114 L115 L116 L117 | L118 L119 L120 L121 | L122 L123 L124 L125 | L131 L130 L129 L128 | L132 L133 L134 L135 | L136 L137 L138 L139 | L140 L141 L142 L143 | L144 L145 L146 L147 | L151 L150 L149 L148 | L155 L154 L153 L152 | L159 L158 L157 L156 | L163 L162 L161 L160 | L164 L165 L166 L167 | L171 L170 L169 L168 | L254 L174 L173 L172 | L255 L177 L176 L175 | L181 L180 L179 L178 | L182 L183 L184 L185 | L189 L188 L187 L186 | L190 L191 L192 L193 | L197 L196 L195 L194 | L198 L199 L200 L201 | L205 L204 L203 L202 | L209 L208 L207 L206 | L210 L211 L212 L213 | L214 L215 L216 L217 | L218 L219 L220 L221 | L225 L224 L223 L222 | L226 L227 L228 L229 | L230 L231 L232 L233 | L234 L235 L236 L237 | L241 L240 L239 L238 | L245 L244 L243 L242 | L249 L248 L247 L246 | L253 L252 L251 L250 | L277 L278 L279 L276 | L281 L282 L283 L280 | L289 L290 L291 L288 | L341 L342 L343 L340 | L357 L358 L359 L356 | L365 L366 L367 L364 | L369 L370 L371 L368 | L377 L378 L379 L376 | L409 L410 L411 L408 | L429 L430 L431 L428 | L437 L438 L439 L436 | L449 L450 L451 L448 | L473 L474 L475 L472 | L513 L514 L515 L512
sketch "Sketch2" plane through (0, 0, 7) normal (0, 0, 1) x (1, 0, 0)
  line L0 (1.062, 1.062) -> (1.062, 7.062) projected
  line L1 (1.062, 1.062) -> (7.062, 1.062)
  line L2 (7.062, 1.062) -> (7.062, 7.062)
  line L3 (7.062, 7.062) -> (1.062, 7.062)
  line L4 (1.062, 7.062) -> (1.062, 1.062)
  line L5 (6.562, 1.562) -> (1.562, 1.562)
  line L6 (1.562, 1.562) -> (1.562, 6.562)
  line L7 (1.562, 6.562) -> (6.562, 6.562)
  line L8 (6.562, 6.562) -> (6.562, 1.562)
  line L9 (1.062, 9.186) -> (7.062, 9.186)
  line L10 (1.062, 15.186) -> (1.062, 9.186)
  line L11 (7.062, 15.186) -> (1.062, 15.186)
  line L12 (7.062, 9.186) -> (7.062, 15.186)
  line L13 (6.562, 14.686) -> (6.562, 9.686)
  line L14 (6.562, 9.686) -> (1.562, 9.686)
  line L15 (1.562, 9.686) -> (1.562, 14.686)
  line L16 (1.562, 14.686) -> (6.562, 14.686)
  line L17 (1.062, 17.31) -> (7.062, 17.31)
  line L18 (1.062, 23.31) -> (1.062, 17.31)
  line L19 (7.062, 23.31) -> (1.062, 23.31)
  line L20 (7.062, 17.31) -> (7.062, 23.31)
  line L21 (6.562, 22.81) -> (6.562, 17.81)
  line L22 (6.562, 17.81) -> (1.562, 17.81)
  line L23 (1.562, 17.81) -> (1.562, 22.81)
  line L24 (1.562, 22.81) -> (6.562, 22.81)
  line L25 (1.062, 25.434) -> (7.062, 25.434)
  line L26 (1.062, 31.434) -> (1.062, 25.434)
  line L27 (7.062, 31.434) -> (1.062, 31.434)
  line L28 (7.062, 25.434) -> (7.062, 31.434)
  line L29 (6.562, 30.934) -> (6.562, 25.934)
  line L30 (6.562, 25.934) -> (1.562, 25.934)
  line L31 (1.562, 25.934) -> (1.562, 30.934)
  line L32 (1.562, 30.934) -> (6.562, 30.934)
  line L33 (1.062, 33.558) -> (7.062, 33.558)
  line L34 (1.062, 39.558) -> (1.062, 33.558)
  line L35 (7.062, 39.558) -> (1.062, 39.558)
  line L36 (7.062, 33.558) -> (7.062, 39.558)
  line L37 (6.562, 39.058) -> (6.562, 34.058)
  line L38 (6.562, 34.058) -> (1.562, 34.058)
  line L39 (1.562, 34.058) -> (1.562, 39.058)
  line L40 (1.562, 39.058) -> (6.562, 39.058)
  line L41 (1.062, 41.682) -> (7.062, 41.682)
  line L42 (1.062, 47.682) -> (1.062, 41.682)
  line L43 (7.062, 47.682) -> (1.062, 47.682)
  line L44 (7.062, 41.682) -> (7.062, 47.682)
  line L45 (6.562, 47.182) -> (6.562, 42.182)
  line L46 (6.562, 42.182) -> (1.562, 42.182)
  line L47 (1.562, 42.182) -> (1.562, 47.182)
  line L48 (1.562, 47.182) -> (6.562, 47.182)
  line L49 (1.062, 49.806) -> (7.062, 49.806)
  line L50 (1.062, 55.806) -> (1.062, 49.806)
  line L51 (7.062, 55.806) -> (1.062, 55.806)
  line L52 (7.062, 49.806) -> (7.062, 55.806)
  line L53 (6.562, 55.306) -> (6.562, 50.306)
  line L54 (6.562, 50.306) -> (1.562, 50.306)
  line L55 (1.562, 50.306) -> (1.562, 55.306)
  line L56 (1.562, 55.306) -> (6.562, 55.306)
  line L57 (1.062, 57.93) -> (7.062, 57.93)
  line L58 (1.062, 63.93) -> (1.062, 57.93)
  line L59 (7.062, 63.93) -> (1.062, 63.93)
  line L60 (7.062, 57.93) -> (7.062, 63.93)
  line L61 (6.562, 63.43) -> (6.562, 58.43)
  line L62 (6.562, 58.43) -> (1.562, 58.43)
  line L63 (1.562, 58.43) -> (1.562, 63.43)
  line L64 (1.562, 63.43) -> (6.562, 63.43)
  line L65 (9.186, 1.062) -> (15.186, 1.062)
  line L66 (9.186, 7.062) -> (9.186, 1.062)
  line L67 (15.186, 7.062) -> (9.186, 7.062)
  line L68 (15.186, 1.062) -> (15.186, 7.062)
  line L69 (14.686, 6.562) -> (14.686, 1.562)
  line L70 (14.686, 1.562) -> (9.686, 1.562)
  line L71 (9.686, 1.562) -> (9.686, 6.562)
  line L72 (9.686, 6.562) -> (14.686, 6.562)
  line L73 (9.186, 9.186) -> (15.186, 9.186)
  line L74 (9.186, 15.186) -> (9.186, 9.186)
  line L75 (15.186, 15.186) -> (9.186, 15.186)
  line L76 (15.186, 9.186) -> (15.186, 15.186)
  line L77 (14.686, 14.686) -> (14.686, 9.686)
  line L78 (14.686, 9.686) -> (9.686, 9.686)
  line L79 (9.686, 9.686) -> (9.686, 14.686)
  line L80 (9.686, 14.686) -> (14.686, 14.686)
  line L81 (9.186, 17.31) -> (15.186, 17.31)
  line L82 (9.186, 23.31) -> (9.186, 17.31)
  line L83 (15.186, 23.31) -> (9.186, 23.31)
  line L84 (15.186, 17.31) -> (15.186, 23.31)
  line L85 (14.686, 22.81) -> (14.686, 17.81)
  line L86 (14.686, 17.81) -> (9.686, 17.81)
  line L87 (9.686, 17.81) -> (9.686, 22.81)
  line L88 (9.686, 22.81) -> (14.686, 22.81)
  line L89 (9.186, 25.434) -> (15.186, 25.434)
  line L90 (9.186, 31.434) -> (9.186, 25.434)
  line L91 (15.186, 31.434) -> (9.186, 31.434)
  line L92 (15.186, 25.434) -> (15.186, 31.434)
  line L93 (14.686, 30.934) -> (14.686, 25.934)
  line L94 (14.686, 25.934) -> (9.686, 25.934)
  line L95 (9.686, 25.934) -> (9.686, 30.934)
  line L96 (9.686, 30.934) -> (14.686, 30.934)
  line L97 (9.186, 33.558) -> (15.186, 33.558)
  line L98 (9.186, 39.558) -> (9.186, 33.558)
  line L99 (15.186, 39.558) -> (9.186, 39.558)
  line L100 (15.186, 33.558) -> (15.186, 39.558)
  line L101 (14.686, 39.058) -> (14.686, 34.058)
  line L102 (14.686, 34.058) -> (9.686, 34.058)
  line L103 (9.686, 34.058) -> (9.686, 39.058)
  line L104 (9.686, 39.058) -> (14.686, 39.058)
  line L105 (9.186, 41.682) -> (15.186, 41.682)
  line L106 (9.186, 47.682) -> (9.186, 41.682)
  line L107 (15.186, 47.682) -> (9.186, 47.682)
  line L108 (15.186, 41.682) -> (15.186, 47.682)
  line L109 (14.686, 47.182) -> (14.686, 42.182)
  line L110 (14.686, 42.182) -> (9.686, 42.182)
  line L111 (9.686, 42.182) -> (9.686, 47.182)
  line L112 (9.686, 47.182) -> (14.686, 47.182)
  line L113 (9.186, 49.806) -> (15.186, 49.806)
  line L114 (9.186, 55.806) -> (9.186, 49.806)
  line L115 (15.186, 55.806) -> (9.186, 55.806)
  line L116 (15.186, 49.806) -> (15.186, 55.806)
  line L117 (14.686, 55.306) -> (14.686, 50.306)
  line L118 (14.686, 50.306) -> (9.686, 50.306)
  line L119 (9.686, 50.306) -> (9.686, 55.306)
  line L120 (9.686, 55.306) -> (14.686, 55.306)
  line L121 (9.186, 57.93) -> (15.186, 57.93)
  line L122 (9.186, 63.93) -> (9.186, 57.93)
  line L123 (15.186, 63.93) -> (9.186, 63.93)
  line L124 (15.186, 57.93) -> (15.186, 63.93)
  line L125 (14.686, 63.43) -> (14.686, 58.43)
  line L126 (14.686, 58.43) -> (9.686, 58.43)
  line L127 (9.686, 58.43) -> (9.686, 63.43)
  line L128 (9.686, 63.43) -> (14.686, 63.43)
  line L129 (17.31, 1.062) -> (23.31, 1.062)
  line L130 (17.31, 7.062) -> (17.31, 1.062)
  line L131 (23.31, 7.062) -> (17.31, 7.062)
  line L132 (23.31, 1.062) -> (23.31, 7.062)
  line L133 (22.81, 6.562) -> (22.81, 1.562)
  line L134 (22.81, 1.562) -> (17.81, 1.562)
  line L135 (17.81, 1.562) -> (17.81, 6.562)
  line L136 (17.81, 6.562) -> (22.81, 6.562)
  line L137 (17.31, 9.186) -> (23.31, 9.186)
  line L138 (17.31, 15.186) -> (17.31, 9.186)
  line L139 (23.31, 15.186) -> (17.31, 15.186)
  line L140 (23.31, 9.186) -> (23.31, 15.186)
  line L141 (22.81, 14.686) -> (22.81, 9.686)
  line L142 (22.81, 9.686) -> (17.81, 9.686)
  line L143 (17.81, 9.686) -> (17.81, 14.686)
  line L144 (17.81, 14.686) -> (22.81, 14.686)
  line L145 (17.31, 17.31) -> (23.31, 17.31)
  line L146 (17.31, 23.31) -> (17.31, 17.31)
  line L147 (23.31, 23.31) -> (17.31, 23.31)
  line L148 (23.31, 17.31) -> (23.31, 23.31)
  line L149 (22.81, 22.81) -> (22.81, 17.81)
  line L150 (22.81, 17.81) -> (17.81, 17.81)
  line L151 (17.81, 17.81) -> (17.81, 22.81)
  line L152 (17.81, 22.81) -> (22.81, 22.81)
  line L153 (17.31, 25.434) -> (23.31, 25.434)
  line L154 (17.31, 31.434) -> (17.31, 25.434)
  line L155 (23.31, 31.434) -> (17.31, 31.434)
  line L156 (23.31, 25.434) -> (23.31, 31.434)
  line L157 (22.81, 30.934) -> (22.81, 25.934)
  line L158 (22.81, 25.934) -> (17.81, 25.934)
  line L159 (17.81, 25.934) -> (17.81, 30.934)
  line L160 (17.81, 30.934) -> (22.81, 30.934)
  line L161 (17.31, 33.558) -> (23.31, 33.558)
  line L162 (17.31, 39.558) -> (17.31, 33.558)
  line L163 (23.31, 39.558) -> (17.31, 39.558)
  line L164 (23.31, 33.558) -> (23.31, 39.558)
  line L165 (22.81, 39.058) -> (22.81, 34.058)
  line L166 (22.81, 34.058) -> (17.81, 34.058)
  line L167 (17.81, 34.058) -> (17.81, 39.058)
  line L168 (17.81, 39.058) -> (22.81, 39.058)
  line L169 (17.31, 41.682) -> (23.31, 41.682)
  line L170 (17.31, 47.682) -> (17.31, 41.682)
  line L171 (23.31, 47.682) -> (17.31, 47.682)
  line L172 (23.31, 41.682) -> (23.31, 47.682)
  line L173 (22.81, 47.182) -> (22.81, 42.182)
  line L174 (22.81, 42.182) -> (17.81, 42.182)
  line L175 (17.81, 42.182) -> (17.81, 47.182)
  line L176 (17.81, 47.182) -> (22.81, 47.182)
  line L177 (17.31, 49.806) -> (23.31, 49.806)
  line L178 (17.31, 55.806) -> (17.31, 49.806)
  line L179 (23.31, 55.806) -> (17.31, 55.806)
  line L180 (23.31, 49.806) -> (23.31, 55.806)
  line L181 (22.81, 55.306) -> (22.81, 50.306)
  line L182 (22.81, 50.306) -> (17.81, 50.306)
  line L183 (17.81, 50.306) -> (17.81, 55.306)
  line L184 (17.81, 55.306) -> (22.81, 55.306)
  line L185 (17.31, 57.93) -> (23.31, 57.93)
  line L186 (17.31, 63.93) -> (17.31, 57.93)
  line L187 (23.31, 63.93) -> (17.31, 63.93)
  line L188 (23.31, 57.93) -> (23.31, 63.93)
  line L189 (22.81, 63.43) -> (22.81, 58.43)
  line L190 (22.81, 58.43) -> (17.81, 58.43)
  line L191 (17.81, 58.43) -> (17.81, 63.43)
  line L192 (17.81, 63.43) -> (22.81, 63.43)
  line L193 (25.434, 1.062) -> (31.434, 1.062)
  line L194 (25.434, 7.062) -> (25.434, 1.062)
  line L195 (31.434, 7.062) -> (25.434, 7.062)
  line L196 (31.434, 1.062) -> (31.434, 7.062)
  line L197 (30.934, 6.562) -> (30.934, 1.562)
  line L198 (30.934, 1.562) -> (25.934, 1.562)
  line L199 (25.934, 1.562) -> (25.934, 6.562)
  line L200 (25.934, 6.562) -> (30.934, 6.562)
  line L201 (25.434, 9.186) -> (31.434, 9.186)
  line L202 (25.434, 15.186) -> (25.434, 9.186)
  line L203 (31.434, 15.186) -> (25.434, 15.186)
  line L204 (31.434, 9.186) -> (31.434, 15.186)
  line L205 (30.934, 14.686) -> (30.934, 9.686)
  line L206 (30.934, 9.686) -> (25.934, 9.686)
  line L207 (25.934, 9.686) -> (25.934, 14.686)
  line L208 (25.934, 14.686) -> (30.934, 14.686)
  line L209 (25.434, 17.31) -> (31.434, 17.31)
  line L210 (25.434, 23.31) -> (25.434, 17.31)
  line L211 (31.434, 23.31) -> (25.434, 23.31)
  line L212 (31.434, 17.31) -> (31.434, 23.31)
  line L213 (30.934, 22.81) -> (30.934, 17.81)
  line L214 (30.934, 17.81) -> (25.934, 17.81)
  line L215 (25.934, 17.81) -> (25.934, 22.81)
  line L216 (25.934, 22.81) -> (30.934, 22.81)
  line L217 (25.434, 25.434) -> (31.434, 25.434)
  line L218 (25.434, 31.434) -> (25.434, 25.434)
  line L219 (31.434, 31.434) -> (25.434, 31.434)
  line L220 (31.434, 25.434) -> (31.434, 31.434)
  line L221 (30.934, 30.934) -> (30.934, 25.934)
  line L222 (30.934, 25.934) -> (25.934, 25.934)
  line L223 (25.934, 25.934) -> (25.934, 30.934)
  line L224 (25.934, 30.934) -> (30.934, 30.934)
  line L225 (25.434, 33.558) -> (31.434, 33.558)
  line L226 (25.434, 39.558) -> (25.434, 33.558)
  line L227 (31.434, 39.558) -> (25.434, 39.558)
  line L228 (31.434, 33.558) -> (31.434, 39.558)
  line L229 (30.934, 39.058) -> (30.934, 34.058)
  line L230 (30.934, 34.058) -> (25.934, 34.058)
  line L231 (25.934, 34.058) -> (25.934, 39.058)
  line L232 (25.934, 39.058) -> (30.934, 39.058)
  line L233 (25.434, 41.682) -> (31.434, 41.682)
  line L234 (25.434, 47.682) -> (25.434, 41.682)
  line L235 (31.434, 47.682) -> (25.434, 47.682)
  line L236 (31.434, 41.682) -> (31.434, 47.682)
  line L237 (30.934, 47.182) -> (30.934, 42.182)
  line L238 (30.934, 42.182) -> (25.934, 42.182)
  line L239 (25.934, 42.182) -> (25.934, 47.182)
  line L240 (25.934, 47.182) -> (30.934, 47.182)
  line L241 (25.434, 49.806) -> (31.434, 49.806)
  line L242 (25.434, 55.806) -> (25.434, 49.806)
  line L243 (31.434, 55.806) -> (25.434, 55.806)
  line L244 (31.434, 49.806) -> (31.434, 55.806)
  line L245 (30.934, 55.306) -> (30.934, 50.306)
  line L246 (30.934, 50.306) -> (25.934, 50.306)
  line L247 (25.934, 50.306) -> (25.934, 55.306)
  line L248 (25.934, 55.306) -> (30.934, 55.306)
  line L249 (25.434, 57.93) -> (31.434, 57.93)
  line L250 (25.434, 63.93) -> (25.434, 57.93)
  line L251 (31.434, 63.93) -> (25.434, 63.93)
  line L252 (31.434, 57.93) -> (31.434, 63.93)
  line L253 (30.934, 63.43) -> (30.934, 58.43)
  line L254 (30.934, 58.43) -> (25.934, 58.43)
  line L255 (25.934, 58.43) -> (25.934, 63.43)
  line L256 (25.934, 63.43) -> (30.934, 63.43)
  line L257 (33.558, 1.062) -> (39.558, 1.062)
  line L258 (33.558, 7.062) -> (33.558, 1.062)
  line L259 (39.558, 7.062) -> (33.558, 7.062)
  line L260 (39.558, 1.062) -> (39.558, 7.062)
  line L261 (39.058, 6.562) -> (39.058, 1.562)
  line L262 (39.058, 1.562) -> (34.058, 1.562)
  line L263 (34.058, 1.562) -> (34.058, 6.562)
  line L264 (34.058, 6.562) -> (39.058, 6.562)
  line L265 (33.558, 9.186) -> (39.558, 9.186)
  line L266 (33.558, 15.186) -> (33.558, 9.186)
  line L267 (39.558, 15.186) -> (33.558, 15.186)
  line L268 (39.558, 9.186) -> (39.558, 15.186)
  line L269 (39.058, 14.686) -> (39.058, 9.686)
  line L270 (39.058, 9.686) -> (34.058, 9.686)
  line L271 (34.058, 9.686) -> (34.058, 14.686)
  line L272 (34.058, 14.686) -> (39.058, 14.686)
  line L273 (33.558, 17.31) -> (39.558, 17.31)
  line L274 (33.558, 23.31) -> (33.558, 17.31)
  line L275 (39.558, 23.31) -> (33.558, 23.31)
  line L276 (39.558, 17.31) -> (39.558, 23.31)
  line L277 (39.058, 22.81) -> (39.058, 17.81)
  line L278 (39.058, 17.81) -> (34.058, 17.81)
  line L279 (34.058, 17.81) -> (34.058, 22.81)
  line L280 (34.058, 22.81) -> (39.058, 22.81)
  line L281 (33.558, 25.434) -> (39.558, 25.434)
  line L282 (33.558, 31.434) -> (33.558, 25.434)
  line L283 (39.558, 31.434) -> (33.558, 31.434)
  line L284 (39.558, 25.434) -> (39.558, 31.434)
  line L285 (39.058, 30.934) -> (39.058, 25.934)
  line L286 (39.058, 25.934) -> (34.058, 25.934)
  line L287 (34.058, 25.934) -> (34.058, 30.934)
  line L288 (34.058, 30.934) -> (39.058, 30.934)
  line L289 (33.558, 33.558) -> (39.558, 33.558)
  line L290 (33.558, 39.558) -> (33.558, 33.558)
  line L291 (39.558, 39.558) -> (33.558, 39.558)
  line L292 (39.558, 33.558) -> (39.558, 39.558)
  line L293 (39.058, 39.058) -> (39.058, 34.058)
  line L294 (39.058, 34.058) -> (34.058, 34.058)
  line L295 (34.058, 34.058) -> (34.058, 39.058)
  line L296 (34.058, 39.058) -> (39.058, 39.058)
  line L297 (33.558, 41.682) -> (39.558, 41.682)
  line L298 (33.558, 47.682) -> (33.558, 41.682)
  line L299 (39.558, 47.682) -> (33.558, 47.682)
  line L300 (39.558, 41.682) -> (39.558, 47.682)
  line L301 (39.058, 47.182) -> (39.058, 42.182)
  line L302 (39.058, 42.182) -> (34.058, 42.182)
  line L303 (34.058, 42.182) -> (34.058, 47.182)
  line L304 (34.058, 47.182) -> (39.058, 47.182)
  line L305 (33.558, 49.806) -> (39.558, 49.806)
  line L306 (33.558, 55.806) -> (33.558, 49.806)
  line L307 (39.558, 55.806) -> (33.558, 55.806)
  line L308 (39.558, 49.806) -> (39.558, 55.806)
  line L309 (39.058, 55.306) -> (39.058, 50.306)
  line L310 (39.058, 50.306) -> (34.058, 50.306)
  line L311 (34.058, 50.306) -> (34.058, 55.306)
  line L312 (34.058, 55.306) -> (39.058, 55.306)
  line L313 (33.558, 57.93) -> (39.558, 57.93)
  line L314 (33.558, 63.93) -> (33.558, 57.93)
  line L315 (39.558, 63.93) -> (33.558, 63.93)
  line L316 (39.558, 57.93) -> (39.558, 63.93)
  line L317 (39.058, 63.43) -> (39.058, 58.43)
  line L318 (39.058, 58.43) -> (34.058, 58.43)
  line L319 (34.058, 58.43) -> (34.058, 63.43)
  line L320 (34.058, 63.43) -> (39.058, 63.43)
  line L321 (41.682, 1.062) -> (47.682, 1.062)
  line L322 (41.682, 7.062) -> (41.682, 1.062)
  line L323 (47.682, 7.062) -> (41.682, 7.062)
  line L324 (47.682, 1.062) -> (47.682, 7.062)
  line L325 (47.182, 6.562) -> (47.182, 1.562)
  line L326 (47.182, 1.562) -> (42.182, 1.562)
  line L327 (42.182, 1.562) -> (42.182, 6.562)
  line L328 (42.182, 6.562) -> (47.182, 6.562)
  line L329 (41.682, 9.186) -> (47.682, 9.186)
  line L330 (41.682, 15.186) -> (41.682, 9.186)
  line L331 (47.682, 15.186) -> (41.682, 15.186)
  line L332 (47.682, 9.186) -> (47.682, 15.186)
  line L333 (47.182, 14.686) -> (47.182, 9.686)
  line L334 (47.182, 9.686) -> (42.182, 9.686)
  line L335 (42.182, 9.686) -> (42.182, 14.686)
  line L336 (42.182, 14.686) -> (47.182, 14.686)
  line L337 (41.682, 17.31) -> (47.682, 17.31)
  line L338 (41.682, 23.31) -> (41.682, 17.31)
  line L339 (47.682, 23.31) -> (41.682, 23.31)
  line L340 (47.682, 17.31) -> (47.682, 23.31)
  line L341 (47.182, 22.81) -> (47.182, 17.81)
  line L342 (47.182, 17.81) -> (42.182, 17.81)
  line L343 (42.182, 17.81) -> (42.182, 22.81)
  line L344 (42.182, 22.81) -> (47.182, 22.81)
  line L345 (41.682, 25.434) -> (47.682, 25.434)
  line L346 (41.682, 31.434) -> (41.682, 25.434)
  line L347 (47.682, 31.434) -> (41.682, 31.434)
  line L348 (47.682, 25.434) -> (47.682, 31.434)
  line L349 (47.182, 30.934) -> (47.182, 25.934)
  line L350 (47.182, 25.934) -> (42.182, 25.934)
  line L351 (42.182, 25.934) -> (42.182, 30.934)
  line L352 (42.182, 30.934) -> (47.182, 30.934)
  line L353 (41.682, 33.558) -> (47.682, 33.558)
  line L354 (41.682, 39.558) -> (41.682, 33.558)
  line L355 (47.682, 39.558) -> (41.682, 39.558)
  line L356 (47.682, 33.558) -> (47.682, 39.558)
  line L357 (47.182, 39.058) -> (47.182, 34.058)
  line L358 (47.182, 34.058) -> (42.182, 34.058)
  line L359 (42.182, 34.058) -> (42.182, 39.058)
  line L360 (42.182, 39.058) -> (47.182, 39.058)
  line L361 (41.682, 41.682) -> (47.682, 41.682)
  line L362 (41.682, 47.682) -> (41.682, 41.682)
  line L363 (47.682, 47.682) -> (41.682, 47.682)
  line L364 (47.682, 41.682) -> (47.682, 47.682)
  line L365 (47.182, 47.182) -> (47.182, 42.182)
  line L366 (47.182, 42.182) -> (42.182, 42.182)
  line L367 (42.182, 42.182) -> (42.182, 47.182)
  line L368 (42.182, 47.182) -> (47.182, 47.182)
  line L369 (41.682, 49.806) -> (47.682, 49.806)
  line L370 (41.682, 55.806) -> (41.682, 49.806)
  line L371 (47.682, 55.806) -> (41.682, 55.806)
  line L372 (47.682, 49.806) -> (47.682, 55.806)
  line L373 (47.182, 55.306) -> (47.182, 50.306)
  line L374 (47.182, 50.306) -> (42.182, 50.306)
  line L375 (42.182, 50.306) -> (42.182, 55.306)
  line L376 (42.182, 55.306) -> (47.182, 55.306)
  line L377 (41.682, 57.93) -> (47.682, 57.93)
  line L378 (41.682, 63.93) -> (41.682, 57.93)
  line L379 (47.682, 63.93) -> (41.682, 63.93)
  line L380 (47.682, 57.93) -> (47.682, 63.93)
  line L381 (47.182, 63.43) -> (47.182, 58.43)
  line L382 (47.182, 58.43) -> (42.182, 58.43)
  line L383 (42.182, 58.43) -> (42.182, 63.43)
  line L384 (42.182, 63.43) -> (47.182, 63.43)
  line L385 (49.806, 1.062) -> (55.806, 1.062)
  line L386 (49.806, 7.062) -> (49.806, 1.062)
  line L387 (55.806, 7.062) -> (49.806, 7.062)
  line L388 (55.806, 1.062) -> (55.806, 7.062)
  line L389 (55.306, 6.562) -> (55.306, 1.562)
  line L390 (55.306, 1.562) -> (50.306, 1.562)
  line L391 (50.306, 1.562) -> (50.306, 6.562)
  line L392 (50.306, 6.562) -> (55.306, 6.562)
  line L393 (49.806, 9.186) -> (55.806, 9.186)
  line L394 (49.806, 15.186) -> (49.806, 9.186)
  line L395 (55.806, 15.186) -> (49.806, 15.186)
  line L396 (55.806, 9.186) -> (55.806, 15.186)
  line L397 (55.306, 14.686) -> (55.306, 9.686)
  line L398 (55.306, 9.686) -> (50.306, 9.686)
  line L399 (50.306, 9.686) -> (50.306, 14.686)
  line L400 (50.306, 14.686) -> (55.306, 14.686)
  line L401 (49.806, 17.31) -> (55.806, 17.31)
  line L402 (49.806, 23.31) -> (49.806, 17.31)
  line L403 (55.806, 23.31) -> (49.806, 23.31)
  line L404 (55.806, 17.31) -> (55.806, 23.31)
  line L405 (55.306, 22.81) -> (55.306, 17.81)
  line L406 (55.306, 17.81) -> (50.306, 17.81)
  line L407 (50.306, 17.81) -> (50.306, 22.81)
  line L408 (50.306, 22.81) -> (55.306, 22.81)
  line L409 (49.806, 25.434) -> (55.806, 25.434)
  line L410 (49.806, 31.434) -> (49.806, 25.434)
  line L411 (55.806, 31.434) -> (49.806, 31.434)
  line L412 (55.806, 25.434) -> (55.806, 31.434)
  line L413 (55.306, 30.934) -> (55.306, 25.934)
  line L414 (55.306, 25.934) -> (50.306, 25.934)
  line L415 (50.306, 25.934) -> (50.306, 30.934)
  line L416 (50.306, 30.934) -> (55.306, 30.934)
  line L417 (49.806, 33.558) -> (55.806, 33.558)
  line L418 (49.806, 39.558) -> (49.806, 33.558)
  line L419 (55.806, 39.558) -> (49.806, 39.558)
  line L420 (55.806, 33.558) -> (55.806, 39.558)
  line L421 (55.306, 39.058) -> (55.306, 34.058)
  line L422 (55.306, 34.058) -> (50.306, 34.058)
  line L423 (50.306, 34.058) -> (50.306, 39.058)
  line L424 (50.306, 39.058) -> (55.306, 39.058)
  line L425 (49.806, 41.682) -> (55.806, 41.682)
  line L426 (49.806, 47.682) -> (49.806, 41.682)
  line L427 (55.806, 47.682) -> (49.806, 47.682)
  line L428 (55.806, 41.682) -> (55.806, 47.682)
  line L429 (55.306, 47.182) -> (55.306, 42.182)
  line L430 (55.306, 42.182) -> (50.306, 42.182)
  line L431 (50.306, 42.182) -> (50.306, 47.182)
  line L432 (50.306, 47.182) -> (55.306, 47.182)
  line L433 (49.806, 49.806) -> (55.806, 49.806)
  line L434 (49.806, 55.806) -> (49.806, 49.806)
  line L435 (55.806, 55.806) -> (49.806, 55.806)
  line L436 (55.806, 49.806) -> (55.806, 55.806)
  line L437 (55.306, 55.306) -> (55.306, 50.306)
  line L438 (55.306, 50.306) -> (50.306, 50.306)
  line L439 (50.306, 50.306) -> (50.306, 55.306)
  line L440 (50.306, 55.306) -> (55.306, 55.306)
  line L441 (49.806, 57.93) -> (55.806, 57.93)
  line L442 (49.806, 63.93) -> (49.806, 57.93)
  line L443 (55.806, 63.93) -> (49.806, 63.93)
  line L444 (55.806, 57.93) -> (55.806, 63.93)
  line L445 (55.306, 63.43) -> (55.306, 58.43)
  line L446 (55.306, 58.43) -> (50.306, 58.43)
  line L447 (50.306, 58.43) -> (50.306, 63.43)
  line L448 (50.306, 63.43) -> (55.306, 63.43)
  line L449 (57.93, 1.062) -> (63.93, 1.062)